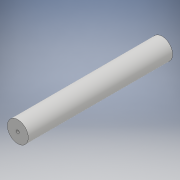
# Autodesk Inventor part: Вал
Saved by Autodesk Inventor 2018 (Build 220112000, 112)
## iProperties
Created: 2023-01-16
Part Number: Вал
Material: Типовые
Document SubType Name: Modeling
Designer: exper
Density: 1 g/cm^3
Appearance: По умолчанию
Author: exper
## iProperties of the stored document Вал_3DПЕЧАТЬ.ipt
Created: 2023-01-16
Part Number: Вал_3DПЕЧАТЬ
Material: Типовые
Document SubType Name: Modeling
Designer: exper
Density: 1 g/cm^3
Appearance: По умолчанию
Author: exper
Autodesk Inventor part; units mm, degrees
ref_plane "YZ Plane" through (0, 0, 0) normal (1, 0, 0) x (0, 1, 0)
ref_plane "XZ Plane" through (0, 0, 0) normal (0, 1, 0) x (-1, 0, 0)
ref_plane "XY Plane" through (0, 0, 0) normal (0, 0, 1) x (1, 0, 0)
sketch "Эскиз1" plane through (0, 0, 0) normal (0, 1, 0) x (-1, 0, 0)
  circle A0 centre (0, 0) radius 10.5
  dimension "d0" = 21
  constraints: 1 centre point, 1 coincident
  measures "d0" diameter of A0
extrude "Выдавливание1" add sketch "Эскиз1" along normal blind 145
sketch "Эскиз2" plane through (0, 145, 0) normal (0, 1, 0) x (1, 0, 0)
  point P0 (0, 0)
  point P1 (0, 0)
  constraints: 1 coincident
hole "Отверстие1" at (0, 145, 0) direction (0, -1, 0) diameter 3 end through all
